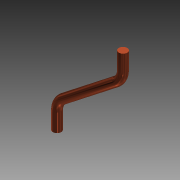
# Autodesk Inventor part: FeedSplitter
Saved by Autodesk Inventor 2014 (Build 180170000, 170)
## iProperties
Created: 2015-05-01
Part Number: FeedSplitter
Material: Generic
Document SubType Name: Modeling
Designer: Owner
Density: 1 g/cm^3
Appearance: Copper - Polished
Author: Owner
Autodesk Inventor part; units mm, degrees
ref_plane "YZ Plane" through (0, 0, 0) normal (1, 0, 0) x (0, 1, 0)
ref_plane "XZ Plane" through (0, 0, 0) normal (0, 1, 0) x (-1, 0, 0)
ref_plane "XY Plane" through (0, 0, 0) normal (0, 0, 1) x (1, 0, 0)
sketch "Sketch1" plane through (0, 0, 0) normal (0, 0, 1) x (1, 0, 0)
  line L0 (0.0306, -0.0332) -> (0.0306, 12.6668)
  line L1 (4.9085, 22.672) -> (44.9292, 53.9606)
  line L2 (49.8071, 63.9658) -> (49.8071, 76.6658)
  arc A0 (4.9085, 22.672) -> (0.0306, 12.6668) centre (12.7306, 12.6668) ccw
  arc A1 (44.9292, 53.9606) -> (49.8071, 63.9658) centre (37.1071, 63.9658) ccw
  point P0 (0, 0)
  point P1 (0.0306, 18.8584)
  dimension "d3" = 12.7
  dimension "d4" = 12.7
  dimension "d5" = 12.7
  dimension "d6" = 50.8
  constraints: 6 end point, 4 point on circle, 4 tangent, 2 centre point, 2 point on line, 1 equal radius, 1 parallel, 1 vertical
  measures "d3" radius of A0
  measures "d4" distance of L0.start L0.end
  measures "d5" distance of L2.start L2.end
  measures "d6" distance of L1.start L1.end
sketch "Sketch2" plane through (0, 0, 0) normal (0, 1, 0) x (-1, 0, 0)
  circle A0 centre (0, 0) radius 3.175
  dimension "d1" = 6.35
  constraints: 1 centre point
  measures "d1" diameter of A0
sweep "Sweep1" add profiles "Sketch2" path "Sketch1" path curves L0 A0 L1 A1 L2
body "Solid1"
